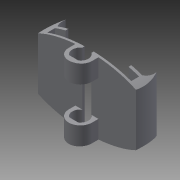
# Autodesk Inventor part: Part2
Saved by Autodesk Inventor 2013 (Build 170138000, 138)
## iProperties
Created: 2013-04-10
Part Number: Part2
Material: Generic
Document SubType Name: Modeling
Designer: Sebastian Saez
Density: 1 g/cm^3
Author: Sebastian Saez
Autodesk Inventor part; units mm, degrees
ref_plane "YZ Plane" through (0, 0, 0) normal (1, 0, 0) x (0, 1, 0)
ref_plane "XZ Plane" through (0, 0, 0) normal (0, 1, 0) x (-1, 0, 0)
ref_plane "XY Plane" through (0, 0, 0) normal (0, 0, 1) x (1, 0, 0)
sketch "Sketch1" plane through (0, 0, 0) normal (0, 1, 0) x (-1, 0, 0)
  arc A0 (-3.4214, 5.0502) -> (-3.422, -5.0498) centre (0, 0) ccw
  line L0 (0.0203, 21.6706) -> (0.0129, -26.6762) construction
  arc A1 (-37.2771, -5.0476) -> (-34.5522, -23.5019) centre (-7.7073, -10.1097) ccw
  line L1 (-3.4222, -6.7364) -> (-31.9825, -6.735)
  line L2 (-23.9829, -14.849) -> (-23.9836, -12.7362)
  line L3 (-23.9829, -14.849) -> (-32.1662, -14.8486)
  line L4 (-40.1598, -25.6638) -> (27.0571, -25.6672) construction
  line L5 (-31.9825, -6.735) -> (-31.9828, -12.735)
  line L6 (-3.422, -5.0498) -> (-3.4222, -6.7364)
  line L7 (0.0182, 6.05) -> (0.0182, 6.05)
  arc A2 (-32.1662, -14.8486) -> (-34.5522, -23.5019) centre (-24.7445, -21.5506) ccw
  line L8 (-8.7772, -5.0495) -> (-37.2771, -5.0476)
  arc A3 (0.0183, 8.7768) -> (-8.7769, 0.0006) centre (0, 0) ccw
  line L9 (-3.4214, 5.0502) -> (0.0178, 5.0497)
  line L10 (24.0123, -14.8564) -> (32.1956, -14.8584)
  arc A4 (34.579, -23.5125) -> (32.1956, -14.8584) centre (24.7718, -21.5582) ccw
  line L11 (24.0123, -14.8564) -> (24.0136, -12.7435)
  line L12 (32.0144, -6.7448) -> (32.0129, -12.7448)
  arc A5 (34.579, -23.5125) -> (37.3096, -5.059) centre (7.7382, -10.1121) ccw
  line L13 (3.4541, -6.7375) -> (32.0144, -6.7448)
  arc A6 (3.4544, -5.0509) -> (3.4569, 5.0491) centre (0.034, 0) ccw
  line L14 (3.4544, -5.0509) -> (3.4541, -6.7375)
  line L15 (8.8096, -5.0521) -> (37.3096, -5.059)
  arc A7 (8.8108, -0.0021) -> (0.0183, 8.7768) centre (0.034, 0) ccw
  line L16 (3.4569, 5.0491) -> (0.0178, 5.0497)
  line L17 (-23.9836, -12.7362) -> (-31.9828, -12.735)
  line L18 (32.0129, -12.7448) -> (24.0136, -12.7435)
  line L19 (-8.7769, 0.0006) -> (-8.7772, -5.0495)
  line L20 (8.8108, -0.0021) -> (8.8096, -5.0521)
  point P0 (0, 0)
  point P1 (-7.1788, -5.0496)
  point P2 (7.2112, -5.0518)
  dimension "d1" = 30
  dimension "d2" = 10
  dimension "d5" = 6
  constraints: 42 end point, 17 symmetric about line, 16 point on circle, 8 centre point, 3 coincident, 3 perpendicular, 2 point on line, 1 collinear, 1 tangent, 4 other
  measures "d1" radius of A1
  measures "d2" radius of A2
  measures "d5" distance of L5.start L5.end
extrude "Extrusion1" add sketch "Sketch1" along normal blind 55
sketch "Sketch2" plane through (-3.4569, 0, 5.0491) normal (0.0002, 0, -1) x (-1, 0, -0.0002)
  line L0 (9.4839, 41) -> (-16.3961, 41)
  line L1 (-16.3961, 41) -> (-16.3961, 14)
  line L2 (-16.3961, 14) -> (9.4839, 14)
  line L3 (9.4839, 14) -> (9.4839, 41)
  line L4 (9.4839, 41) -> (-16.3961, 14) construction
  line L5 (-16.3961, 41) -> (9.4839, 14) construction
  point P0 (-3.4561, 0)
  point P1 (-3.4561, 27.5)
  point P2 (-3.4561, 27.5)
  dimension "d8" = 27
  constraints: 12 end point, 3 midpoint, 2 parallel, 1 horizontal, 1 perpendicular, 1 other
  measures "d8" distance of L2.end L0.start
extrude "Extrusion2" cut sketch "Sketch2" along normal blind 10.0875 and the other way blind 8.219
sketch "Sketch3" plane through (-8.8096, 0, -5.0521) normal (-0.0002, 0, 1) x (1, 0, 0.0002)
  line L0 (14.5295, 41) -> (3.0922, 41)
  line L1 (3.0922, 41) -> (3.0922, 14)
  line L2 (3.0922, 14) -> (14.5295, 14)
  line L3 (14.5295, 14) -> (14.5295, 41)
  line L4 (14.5295, 41) -> (3.0922, 14) construction
  line L5 (3.0922, 41) -> (14.5295, 14) construction
  point P0 (8.8108, 0)
  point P1 (8.8108, 27.5)
  point P2 (8.8108, 27.5)
  dimension "d14" = 27
  constraints: 12 end point, 3 midpoint, 2 parallel, 1 horizontal, 1 perpendicular, 1 other
  measures "d14" distance of L0.end L1.end
extrude "Extrusion3" add sketch "Sketch3" against normal up to surface (1.6867 mm away)
sketch "Sketch4" plane through (-8.8096, 0, -5.0521) normal (-0.0002, 0, 1) x (1, 0, 0.0002)
  line L0 (5.3553, 14) -> (5.3553, 41) projected
  line L1 (5.3553, 14) -> (12.2325, 14) projected
  line L2 (12.2325, 41) -> (12.2325, 14) projected
  line L3 (12.2325, 41) -> (5.3553, 41) projected
  ellipse E0 centre (8.8108, 27.5) end of major axis (8.8108, 0) minor radius 54.0722
  point P0 (8.8108, 0)
  constraints: 1 vertical, 1 vertical alignment, 2 other
extrude "Extrusion4" cut sketch "Sketch4" along normal mid plane 48.0375 keep common part
body "Solid1"
